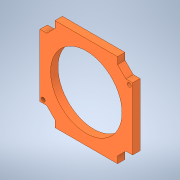
# Autodesk Inventor part: 20_Cube_Insert_CirAp_Guide
Saved by Autodesk Inventor 2022 (Build 260153000, 153)
## iProperties
Created: 2019-10-23
Part Number: 20_Cube_Insert_CirAp_Guide
Material: Generic
Document SubType Name: Modeling
Designer: marsikovabarbora
Density: 1 g/cm^3
Appearance: Default
Author: marsikovabarbora
Autodesk Inventor part; units mm, degrees
ref_plane "YZ Plane" through (0, 0, 0) normal (1, 0, 0) x (0, 1, 0)
ref_plane "XZ Plane" through (0, 0, 0) normal (0, 1, 0) x (-1, 0, 0)
ref_plane "XY Plane" through (0, 0, 0) normal (0, 0, 1) x (1, 0, 0)
sketch "Sketch1" plane through (0, 0, 0) normal (0, 0, 1) x (1, 0, 0)
  line L0 (-34.8609, 0) -> (34.8609, 0) construction
  line L1 (0, -34.8609) -> (0, 34.8609) construction
  line L2 (0, 0) -> (11.6542, 11.6542) construction
  line L3 (0, 0) -> (16.4815, 0) construction
  line L4 (0, 24.9006) -> (16.8, 24.9006)
  line L5 (16.8, 24.9006) -> (16.8, 21.2406)
  line L6 (16.8, 21.2406) -> (19.0203, 19.0203)
  line L7 (24.9006, 0) -> (24.9006, 16.8)
  line L8 (24.9006, 16.8) -> (21.2406, 16.8)
  line L9 (21.2406, 16.8) -> (19.0203, 19.0203)
  line L10 (0, 0) -> (-11.6542, 11.6542) construction
  line L11 (0, 0) -> (-16.4815, 0) construction
  line L12 (0, 24.9006) -> (-16.8, 24.9006)
  line L13 (-16.8, 24.9006) -> (-16.8, 21.2406)
  line L14 (-16.8, 21.2406) -> (-19.0203, 19.0203)
  line L15 (-24.9006, 0) -> (-24.9006, 16.8)
  line L16 (-24.9006, 16.8) -> (-21.2406, 16.8)
  line L17 (-21.2406, 16.8) -> (-19.0203, 19.0203)
  line L18 (0, 0) -> (11.6542, -11.6542) construction
  line L19 (0, -24.9006) -> (16.8, -24.9006)
  line L20 (16.8, -24.9006) -> (16.8, -21.2406)
  line L21 (16.8, -21.2406) -> (19.0203, -19.0203)
  line L22 (24.9006, 0) -> (24.9006, -16.8)
  line L23 (24.9006, -16.8) -> (21.2406, -16.8)
  line L24 (21.2406, -16.8) -> (19.0203, -19.0203)
  line L25 (0, 0) -> (-11.6542, -11.6542) construction
  line L26 (0, -24.9006) -> (-16.8, -24.9006)
  line L27 (-16.8, -24.9006) -> (-16.8, -21.2406)
  line L28 (-16.8, -21.2406) -> (-19.0203, -19.0203)
  line L29 (-24.9006, 0) -> (-24.9006, -16.8)
  line L30 (-24.9006, -16.8) -> (-21.2406, -16.8)
  line L31 (-21.2406, -16.8) -> (-19.0203, -19.0203)
  dimension "d0" = 45
  dimension "d1" = 3.14
  dimension "d2" = 3.66
  dimension "d3" = 16.8
  constraints: 60 end point, 24 symmetric about line, 5 point on line, 2 horizontal, 2 perpendicular, 1 equal length
  measures "d0" angle of L3 L2
  measures "d1" distance of L5.end L6.end
  measures "d2" distance of L4.end L5.end
  measures "d3" distance of L4.start L4.end
extrude "Extrusion1" add sketch "Sketch1" along normal blind 4
hole "Hole1" at (0, 0, 0) direction (0, 0, 1) diameter 40 end through all
sketch "Sketch6" plane through (0, 0, 4) normal (0, 0, 1) x (1, 0, 0)
  circle A0 centre (0, 0) radius 20 construction
  line L0 (16.8, 24.9006) -> (-16.8, 24.9006) construction
  line L1 (-16.8, 24.9006) -> (-16.8, 21.2406) construction
  line L2 (-16.8, 21.2406) -> (-21.2406, 16.8) construction
  line L3 (-21.2406, 16.8) -> (-24.9006, 16.8) construction
  line L4 (-24.9006, 16.8) -> (-24.9006, -16.8) construction
  line L5 (-24.9006, -16.8) -> (-21.2406, -16.8) construction
  line L6 (-21.2406, -16.8) -> (-16.8, -21.2406) construction
  line L7 (-16.8, -21.2406) -> (-16.8, -24.9006) construction
  line L8 (-16.8, -24.9006) -> (16.8, -24.9006) construction
  line L9 (16.8, -24.9006) -> (16.8, -21.2406) construction
  line L10 (16.8, -21.2406) -> (21.2406, -16.8) construction
  line L11 (21.2406, -16.8) -> (24.9006, -16.8) construction
  line L12 (24.9006, -16.8) -> (24.9006, 16.8) construction
  line L13 (24.9006, 16.8) -> (21.2406, 16.8) construction
  line L14 (21.2406, 16.8) -> (16.8, 21.2406) construction
  line L15 (16.8, 21.2406) -> (16.8, 24.9006) construction
  circle A1 centre (0, 0) radius 20
  circle A2 centre (0, 0) radius 13.5
  dimension "d42" = 40
  dimension "d43" = 27
  constraints: 2 centre point, 1 coincident, 1 concentric
  measures "d42" diameter of A1
  measures "d43" diameter of A2
extrude "Extrusion4" [suppressed]
sketch "Sketch8" plane through (0, 0, 4) normal (0, 0, 1) x (1, 0, 0)
  line L0 (16.8, 24.9006) -> (-16.8, 24.9006) projected
  line L1 (-16.8, 24.9006) -> (-16.8, 21.2406) projected
  line L2 (-16.8, 21.2406) -> (-21.2406, 16.8) projected
  line L3 (-21.2406, 16.8) -> (-24.9006, 16.8) projected
  line L4 (-24.9006, 16.8) -> (-24.9006, -16.8) projected
  line L5 (-24.9006, -16.8) -> (-21.2406, -16.8) projected
  line L6 (-21.2406, -16.8) -> (-16.8, -21.2406) projected
  line L7 (-16.8, -21.2406) -> (-16.8, -24.9006) projected
  line L8 (-16.8, -24.9006) -> (16.8, -24.9006) projected
  line L9 (16.8, -24.9006) -> (16.8, -21.2406) projected
  line L10 (16.8, -21.2406) -> (21.2406, -16.8) projected
  line L11 (21.2406, -16.8) -> (24.9006, -16.8) projected
  line L12 (24.9006, -16.8) -> (24.9006, 16.8) projected
  line L13 (24.9006, 16.8) -> (21.2406, 16.8) projected
  line L14 (21.2406, 16.8) -> (16.8, 21.2406) projected
  line L15 (16.8, 21.2406) -> (16.8, 24.9006) projected
  line L16 (-23.9006, -15.8) -> (-23.9006, 15.8)
  line L17 (-23.9006, 15.8) -> (-20.8264, 15.8)
  line L18 (-20.8264, 15.8) -> (-15.8, 20.8264)
  line L19 (-15.8, 20.8264) -> (-15.8, 23.9006)
  line L20 (-15.8, 23.9006) -> (15.8, 23.9006)
  line L21 (15.8, 23.9006) -> (15.8, 20.8264)
  line L22 (15.8, 20.8264) -> (20.8264, 15.8)
  line L23 (20.8264, 15.8) -> (23.9006, 15.8)
  line L24 (23.9006, 15.8) -> (23.9006, -15.8)
  line L25 (23.9006, -15.8) -> (20.8264, -15.8)
  line L26 (20.8264, -15.8) -> (15.8, -20.8264)
  line L27 (15.8, -20.8264) -> (15.8, -23.9006)
  line L28 (15.8, -23.9006) -> (-15.8, -23.9006)
  line L29 (-15.8, -23.9006) -> (-15.8, -20.8264)
  line L30 (-15.8, -20.8264) -> (-20.8264, -15.8)
  line L31 (-20.8264, -15.8) -> (-23.9006, -15.8)
  circle A0 centre (0, 0) radius 20 projected
  circle A1 centre (0, 0) radius 19.2
  dimension "d41" = 1
  dimension "d46" = 0.8
  constraints: 32 end point, 1 centre point, 15 other
  measures "d41" distance between parallel lines of L4 L16
  measures "d46" radial gap between concentric circles of A0 A1
extrude "Extrusion6" add sketch "Sketch8" against normal up to surface (4 mm away)
sketch "Sketch9" plane through (0, 0, 0) normal (0, 0, -1) x (-1, 0, 0)
  circle A0 centre (-23.1006, 15) radius 1.05 projected
  circle A1 centre (23.1006, -15) radius 1.05 projected
  point P0 (0, 0)
extrude "Extrusion7" cut sketch "Sketch9" against normal through all
body "Solid1"
